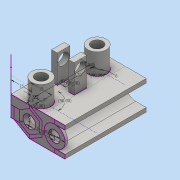
# Autodesk Inventor part: XMountR
Saved by Autodesk Inventor 2016 (Build 200138000, 138)
## iProperties
Created: 2016-09-02
Part Number: XMountR
Material: Generic
Document SubType Name: Modeling
Designer: Sam
Density: 1 g/cm^3
Appearance: Default
Author: Sam
Autodesk Inventor part; units mm, degrees
note: some values were not read from the file. Chosen so that the rebuilt part matches the saved one: direction of "Hole2".
ref_plane "YZ Plane" through (0, 0, 0) normal (1, 0, 0) x (0, 1, 0)
ref_plane "XZ Plane" through (0, 0, 0) normal (0, 1, 0) x (-1, 0, 0)
ref_plane "XY Plane" through (0, 0, 0) normal (0, 0, 1) x (1, 0, 0)
sketch "Sketch1" plane through (0, 0, 0) normal (0, 1, 0) x (-1, 0, 0)
  line L0 (-6.023191, 2.500092) -> (-6.023191, 5.500092) construction
  line L1 (-6.023191, 4.000092) -> (-13.023191, 4.000092) construction
  line L2 (-6.041071, 8.03122) -> (-6.041071, 4.000092)
  line L3 (-6.041071, -0.031037) -> (-13.023191, -4.062166)
  line L4 (-13.023191, -4.062166) -> (-20.005311, -0.031037)
  line L5 (-20.005311, -0.031037) -> (-20.005311, 8.03122)
  line L6 (-20.005311, 8.03122) -> (-13.023191, 12.062349)
  line L7 (-13.023191, 12.062349) -> (-6.041071, 8.03122)
  line L8 (-22.03646, 9.203905) -> (-22.03646, -1.203722)
  line L9 (-22.03646, -1.203722) -> (-13.023191, -6.407535)
  line L10 (-13.023191, 14.407718) -> (-22.03646, 9.203905)
  line L11 (-13.023191, 4.000092) -> (-31.023191, 4.000092) construction
  circle A0 centre (-31.023191, 4.000092) radius 7.5
  line L12 (-13.023191, -6.407535) -> (-30.97685, -6.407535)
  line L13 (-30.97685, -6.407535) -> (-30.97685, -3.499765)
  line L14 (-30.97685, 11.499948) -> (-30.97685, 14.407718)
  line L15 (-30.97685, 14.407718) -> (-13.023191, 14.407718)
  circle A1 centre (-13.023191, 4.000092) radius 4.5
  line L16 (-30.97685, 11.499988) -> (-30.97685, 14.407718)
  line L17 (-30.97685, -3.500012) -> (-30.97685, -6.407535)
  line L18 (-13.023191, -4.062166) -> (-13.023191, -6.407535)
  line L19 (-13.023191, 12.062349) -> (-13.023191, 14.407718)
  line L20 (-6.041071, 4.000092) -> (-6.041071, -0.031037)
  line L21 (-13.023191, 14.407718) -> (0, 14.407718)
  line L22 (0, 39) -> (0, 0)
  line L23 (0, 14.407718) -> (0, 8.03122)
  line L24 (0, 8.03122) -> (-6.041071, 8.03122)
  line L25 (0, 0) -> (-6, 0)
  line L26 (-13.023191, -6.407535) -> (-2, 0)
  line L27 (-2, 0) -> (-2, 8.03122)
  line L28 (-2, 0) -> (0, 0)
  line L29 (0, 8.03122) -> (0, 0)
  circle A2 centre (-31.023191, 4.000092) radius 4
  line L30 (-30.97685, -3.500012) -> (-38.523191, -3.500012)
  line L31 (-38.523191, -3.500012) -> (-38.523191, -6.407535)
  line L32 (-38.523191, -6.407535) -> (-30.97685, -6.407535)
  line L33 (-30.97685, -6.407535) -> (-30.97685, -3.500012)
  line L34 (-30.97685, 14.407718) -> (-38.523191, 14.407718)
  line L35 (-38.523191, 14.407718) -> (-38.523191, 11.499988)
  line L36 (-38.523191, 11.499988) -> (-30.97685, 11.499988)
  line L37 (-30.97685, 11.499988) -> (-30.97685, 14.407718)
  line L38 (0, 26) -> (-15, 26) construction
  point P0 (0, 31)
  dimension "d0" = 7
  dimension "d1" = 18
  dimension "d2" = 15
  dimension "d3" = 9
  dimension "d4" = 8
  dimension "d6" = 15
  constraints: 78 end point, 7 perpendicular, 7 point on line, 6 horizontal, 4 coincident, 4 parallel, 3 centre point, 2 collinear, 2 point on circle, 1 midpoint, 1 vertical, 14 other
  measures "d0" distance of L1.start L1.end
  measures "d1" distance of L11.start L11.end
  measures "d2" diameter of A0
  measures "d3" diameter of A1
  measures "d4" diameter of A2
  measures "d6" distance of L38.start L38.end
extrude "Extrusion1" add sketch "Sketch1" along normal blind 58 contours L24 L27 L26 L18 L3 L20 L2 | L7 L19 L21 L22 L24 | L6 L5 L4 L18 L9 L8 L10 L19 | L24 L22 L25 L27 | L10 L8 L9 L12 L13 A0 L14 L15 | L14 L36 L35 L34 | L32 L31 L30 L13
sketch "Sketch2" plane through (0, 0, 14.407718) normal (0, 0, 1) x (1, 0, 0)
  line L0 (0, 10) -> (15, 10) construction
  line L1 (0, 0) -> (38.523191, 0) construction
  line L2 (15, 0) -> (15, 6.5) construction
  line L3 (15, 0) -> (21.5, 0) construction
  circle A0 centre (15, 6.5) radius 4
  line L4 (15, 6.5) -> (15, 46.5) construction
  line L5 (23.523191, 58) -> (23.523191, 0) construction
  line L6 (15, 6.5) -> (55, 6.5) construction
  circle A1 centre (15, 46.5) radius 4
  circle A2 centre (15, 46.5) radius 6.576473
  circle A3 centre (15, 6.5) radius 6.726812
  line L7 (15, 46.5) -> (15, 26.5) construction
  line L8 (15, 46.5) -> (35, 46.5) construction
  line L9 (15, 26.5) -> (11, 26.5) construction
  line L10 (15, 26.5) -> (19, 26.5) construction
  line L11 (15, 26.5) -> (19, 26.5) construction
  line L12 (7, 31) -> (11, 31)
  line L13 (11, 31) -> (11, 22)
  line L14 (11, 22) -> (7, 22)
  line L15 (7, 22) -> (7, 31)
  line L16 (7, 31) -> (11, 22) construction
  line L17 (11, 31) -> (7, 22) construction
  line L18 (23, 22) -> (19, 22)
  line L19 (19, 22) -> (19, 31)
  line L20 (19, 31) -> (23, 31)
  line L21 (23, 31) -> (23, 22)
  line L22 (23, 22) -> (19, 31) construction
  line L23 (19, 22) -> (23, 31) construction
  point P0 (9, 26.5)
  point P1 (21, 26.5)
  dimension "d9" = 15
  dimension "d10" = 6.5
  dimension "d11" = 90
  dimension "d12" = 8
  dimension "d13" = 40
  dimension "d14" = 90
  dimension "d15" = 8
  dimension "d16" = 2.57647
  dimension "d17" = 2.72681
  dimension "d18" = 20
  dimension "d19" = 90
  dimension "d20" = 4
  dimension "d21" = 180
  constraints: 44 end point, 8 horizontal, 5 parallel, 4 centre point, 4 equal length, 4 midpoint, 3 perpendicular, 3 point on line, 2 coincident, 2 collinear
  measures "d9" distance of L0.start L0.end
  measures "d10" distance of L2.start L2.end
  measures "d11" angle of L3 L2
  measures "d12" diameter of A0
  measures "d13" distance of L4.start L4.end
  measures "d14" angle of L6 L4
  measures "d15" diameter of A1
  measures "d16" radial gap between concentric circles of A1 A2
  measures "d17" radial gap between concentric circles of A0 A3
  measures "d18" distance of L7.start L7.end
  measures "d19" angle of L7 L8
  measures "d20" distance of L7.end L9.end
  measures "d21" angle of L9 L10
extrude "Extrusion2" add sketch "Sketch2" along normal blind 15 contours A2 | A3
extrude "Extrusion3" add sketch "Sketch2" along normal blind 20 contours L12 L13 L14 L15 | L18 L19 L20 L21
hole "Hole1" at (7, 26.5, 28.407718) direction (1, 0, 0) diameter 8 end through all
extrude "Extrusion4" add sketch "Sketch1" along normal blind 4 contours L2 L20 L3 L4 L5 L6 L7
hole "Hole2" at (0, 53, 5) direction (1, 0, 0) diameter 4 end up to surface
sketch "Sketch1 outline for Extrusion5" plane through (0, 0, 0) normal (0, 1, 0) x (-1, 0, 0)
  arc A0 (-30.97685, 11.499948) -> (-30.97685, -3.499765) centre (-31.023191, 4.000092) ccw
  arc A1 (-30.97685, -3.499765) -> (-30.97685, 11.499948) centre (-31.023191, 4.000092) ccw
  circle A2 centre (-31.023191, 4.000092) radius 4
extrude "Extrusion5" add sketch "Sketch1 outline for Extrusion5" along normal blind 2
body "Solid1"
